Autodesk Inventor part; units mm, degrees
(part 3 of 3)
  line L1410 (3.7715, -2.9179) -> (3.7996, -2.8422)
  line L1411 (3.7996, -2.8422) -> (3.7715, -2.9179)
  line L1412 (3.747, -2.9958) -> (3.7715, -2.9179)
  line L1413 (3.7715, -2.9179) -> (3.747, -2.9958)
  line L1414 (3.7261, -3.0758) -> (3.747, -2.9958)
  line L1415 (3.747, -2.9958) -> (3.7261, -3.0758)
  line L1416 (3.7095, -3.158) -> (3.7261, -3.0758)
  line L1417 (3.7261, -3.0758) -> (3.7095, -3.158)
  line L1418 (3.6965, -3.2424) -> (3.7095, -3.158)
  line L1419 (3.7095, -3.158) -> (3.6965, -3.2424)
  line L1420 (3.6879, -3.3289) -> (3.6965, -3.2424)
  line L1421 (3.6965, -3.2424) -> (3.6879, -3.3289)
  line L1422 (3.6828, -3.4176) -> (3.6879, -3.3289)
  line L1423 (3.6879, -3.3289) -> (3.6828, -3.4176)
  line L1424 (3.6814, -3.4911) -> (3.6828, -3.4176)
  line L1425 (3.6828, -3.4176) -> (3.6814, -3.4911)
  line L1426 (3.6843, -3.5899) -> (3.6814, -3.4911)
  line L1427 (3.6814, -3.4911) -> (3.6843, -3.5899)
  line L1428 (3.6944, -3.6821) -> (3.6843, -3.5899)
  line L1429 (3.6843, -3.5899) -> (3.6944, -3.6821)
  line L1430 (3.7102, -3.7687) -> (3.6944, -3.6821)
  line L1431 (3.6944, -3.6821) -> (3.7102, -3.7687)
  line L1432 (3.7326, -3.848) -> (3.7102, -3.7687)
  line L1433 (3.7102, -3.7687) -> (3.7326, -3.848)
  line L1434 (3.7607, -3.9215) -> (3.7326, -3.848)
  line L1435 (3.7326, -3.848) -> (3.7607, -3.9215)
  line L1436 (3.796, -3.9893) -> (3.7607, -3.9215)
  line L1437 (3.7607, -3.9215) -> (3.796, -3.9893)
  line L1438 (3.8371, -4.0498) -> (3.796, -3.9893)
  line L1439 (3.796, -3.9893) -> (3.8371, -4.0498)
  line L1440 (3.8796, -4.0989) -> (3.8371, -4.0498)
  line L1441 (3.8371, -4.0498) -> (3.8796, -4.0989)
  line L1442 (3.9366, -4.1515) -> (3.8796, -4.0989)
  line L1443 (3.8796, -4.0989) -> (3.9366, -4.1515)
  line L1444 (4, -4.1962) -> (3.9366, -4.1515)
  line L1445 (3.9366, -4.1515) -> (4, -4.1962)
  line L1446 (4.0693, -4.2337) -> (4, -4.1962)
  line L1447 (4, -4.1962) -> (4.0693, -4.2337)
  line L1448 (4.1435, -4.2625) -> (4.0693, -4.2337)
  line L1449 (4.0693, -4.2337) -> (4.1435, -4.2625)
  line L1450 (4.2235, -4.2841) -> (4.1435, -4.2625)
  line L1451 (4.1435, -4.2625) -> (4.2235, -4.2841)
  line L1452 (4.3101, -4.2978) -> (4.2235, -4.2841)
  line L1453 (4.2235, -4.2841) -> (4.3101, -4.2978)
  line L1454 (4.4016, -4.3036) -> (4.3101, -4.2978)
  line L1455 (4.3101, -4.2978) -> (4.4016, -4.3036)
  line L1456 (4.4268, -4.3043) -> (4.4016, -4.3036)
  line L1457 (4.4016, -4.3036) -> (4.4268, -4.3043)
  line L1458 (5.4867, -4.2863) -> (5.7138, -3.1998)
  line L1459 (5.7138, -3.1998) -> (5.4867, -4.2863)
  line L1460 (5.4174, -4.3274) -> (5.4867, -4.2863)
  line L1461 (5.4867, -4.2863) -> (5.4174, -4.3274)
  line L1462 (4.5011, -4.3014) -> (4.4268, -4.3043)
  line L1463 (4.4268, -4.3043) -> (4.5011, -4.3014)
  line L1464 (4.5768, -4.2935) -> (4.5011, -4.3014)
  line L1465 (4.5011, -4.3014) -> (4.5768, -4.2935)
  line L1466 (4.6539, -4.2805) -> (4.5768, -4.2935)
  line L1467 (4.5768, -4.2935) -> (4.6539, -4.2805)
  line L1468 (4.7318, -4.2625) -> (4.6539, -4.2805)
  line L1469 (4.6539, -4.2805) -> (4.7318, -4.2625)
  line L1470 (4.8111, -4.2394) -> (4.7318, -4.2625)
  line L1471 (4.7318, -4.2625) -> (4.8111, -4.2394)
  line L1472 (4.8919, -4.2106) -> (4.8111, -4.2394)
  line L1473 (4.8111, -4.2394) -> (4.8919, -4.2106)
  line L1474 (4.9733, -4.1767) -> (4.8919, -4.2106)
  line L1475 (4.8919, -4.2106) -> (4.9733, -4.1767)
  line L1476 (5.0562, -4.1378) -> (4.9733, -4.1767)
  line L1477 (4.9733, -4.1767) -> (5.0562, -4.1378)
  line L1478 (5.1406, -4.0938) -> (5.0562, -4.1378)
  line L1479 (5.0562, -4.1378) -> (5.1406, -4.0938)
  line L1480 (5.1738, -4.0751) -> (5.1406, -4.0938)
  line L1481 (5.1406, -4.0938) -> (5.1738, -4.0751)
  line L1482 (5.2942, -3.5019) -> (5.1738, -4.0751)
  line L1483 (5.1738, -4.0751) -> (5.2942, -3.5019)
  line L1484 (4.4831, -3.5019) -> (5.2942, -3.5019)
  line L1485 (5.2942, -3.5019) -> (4.4831, -3.5019)
  line L1486 (4.5465, -3.1998) -> (4.4831, -3.5019)
  line L1487 (4.4831, -3.5019) -> (4.5465, -3.1998)
  line L1488 (5.7138, -3.1998) -> (4.5465, -3.1998)
  line L1489 (4.5465, -3.1998) -> (5.7138, -3.1998)
  line L1490 (5.6229, -2.1984) -> (5.5717, -2.1379)
  line L1491 (5.5717, -2.1379) -> (5.6229, -2.1984)
  line L1492 (5.6373, -2.2179) -> (5.6229, -2.1984)
  line L1493 (5.6229, -2.1984) -> (5.6373, -2.2179)
  line L1494 (5.677, -2.2813) -> (5.6373, -2.2179)
  line L1495 (5.6373, -2.2179) -> (5.677, -2.2813)
  line L1496 (5.713, -2.3513) -> (5.677, -2.2813)
  line L1497 (5.677, -2.2813) -> (5.713, -2.3513)
  line L1498 (5.7448, -2.427) -> (5.713, -2.3513)
  line L1499 (5.713, -2.3513) -> (5.7448, -2.427)
  line L1500 (5.7721, -2.5092) -> (5.7448, -2.427)
  line L1501 (5.7448, -2.427) -> (5.7721, -2.5092)
  line L1502 (5.7952, -2.5978) -> (5.7721, -2.5092)
  line L1503 (5.7721, -2.5092) -> (5.7952, -2.5978)
  line L1504 (5.8104, -2.667) -> (5.7952, -2.5978)
  line L1505 (5.7952, -2.5978) -> (5.8104, -2.667)
  line L1506 (5.4614, -2.7053) -> (5.8104, -2.667)
  line L1507 (5.8104, -2.667) -> (5.4614, -2.7053)
  line L1508 (5.4383, -2.6159) -> (5.4614, -2.7053)
  line L1509 (5.4614, -2.7053) -> (5.4383, -2.6159)
  line L1510 (5.4088, -2.5337) -> (5.4383, -2.6159)
  line L1511 (5.4383, -2.6159) -> (5.4088, -2.5337)
  line L1512 (5.3727, -2.4587) -> (5.4088, -2.5337)
  line L1513 (5.4088, -2.5337) -> (5.3727, -2.4587)
  line L1514 (5.3288, -2.3909) -> (5.3727, -2.4587)
  line L1515 (5.3727, -2.4587) -> (5.3288, -2.3909)
  line L1516 (5.279, -2.3304) -> (5.3288, -2.3909)
  line L1517 (5.3288, -2.3909) -> (5.279, -2.3304)
  line L1518 (5.2285, -2.2835) -> (5.279, -2.3304)
  line L1519 (5.279, -2.3304) -> (5.2285, -2.2835)
  line L1520 (5.1644, -2.2381) -> (5.2285, -2.2835)
  line L1521 (5.2285, -2.2835) -> (5.1644, -2.2381)
  line L1522 (5.0952, -2.2013) -> (5.1644, -2.2381)
  line L1523 (5.1644, -2.2381) -> (5.0952, -2.2013)
  line L1524 (5.0195, -2.1725) -> (5.0952, -2.2013)
  line L1525 (5.0952, -2.2013) -> (5.0195, -2.1725)
  line L1526 (4.9387, -2.1523) -> (5.0195, -2.1725)
  line L1527 (5.0195, -2.1725) -> (4.9387, -2.1523)
  line L1528 (4.8515, -2.1407) -> (4.9387, -2.1523)
  line L1529 (4.9387, -2.1523) -> (4.8515, -2.1407)
  line L1530 (4.7722, -2.1379) -> (4.8515, -2.1407)
  line L1531 (4.8515, -2.1407) -> (4.7722, -2.1379)
  line L1532 (20, -5.5833) -> (20.6667, -0.5833)
  line L1533 (20, -5.5833) -> (20.6667, -0.5833)
  line L1534 (-20.6667, -5.5833) -> (20, -5.5833)
  line L1535 (-20.6667, -5.5833) -> (20, -5.5833)
  line L1536 (-20, -0.5833) -> (-20.6667, -5.5833)
  line L1537 (-20, -0.5833) -> (-20.6667, -5.5833)
  line L1538 (20.6667, -0.5833) -> (-20, -0.5833)
  line L1539 (20.6667, -0.5833) -> (-20, -0.5833)
  line L1540 (15.8547, -2.1761) -> (15.9643, -2.1797)
  line L1541 (15.9643, -2.1797) -> (15.8547, -2.1761)
  line L1542 (15.9643, -2.1797) -> (16.0551, -2.1869)
  line L1543 (16.0551, -2.1869) -> (15.9643, -2.1797)
  line L1544 (16.0551, -2.1869) -> (16.1265, -2.1984)
  line L1545 (16.1265, -2.1984) -> (16.0551, -2.1869)
  line L1546 (16.1265, -2.1984) -> (16.1799, -2.2143)
  line L1547 (16.1799, -2.2143) -> (16.1265, -2.1984)
  line L1548 (16.1799, -2.2143) -> (16.2022, -2.2251)
  line L1549 (16.2022, -2.2251) -> (16.1799, -2.2143)
  line L1550 (16.2022, -2.2251) -> (16.2707, -2.2727)
  line L1551 (16.2707, -2.2727) -> (16.2022, -2.2251)
  line L1552 (16.2707, -2.2727) -> (16.3233, -2.3361)
  line L1553 (16.3233, -2.3361) -> (16.2707, -2.2727)
  line L1554 (16.3233, -2.3361) -> (16.3457, -2.3801)
  line L1555 (16.3457, -2.3801) -> (16.3233, -2.3361)
  line L1556 (16.3457, -2.3801) -> (16.3673, -2.4587)
  line L1557 (16.3673, -2.4587) -> (16.3457, -2.3801)
  line L1558 (16.3673, -2.4587) -> (16.3745, -2.551)
  line L1559 (16.3745, -2.551) -> (16.3673, -2.4587)
  line L1560 (16.3745, -2.551) -> (16.3745, -2.5539)
  line L1561 (16.3745, -2.5539) -> (16.3745, -2.551)
  line L1562 (16.3745, -2.5539) -> (16.368, -2.6368)
  line L1563 (16.368, -2.6368) -> (16.3745, -2.5539)
  line L1564 (16.368, -2.6368) -> (16.35, -2.7168)
  line L1565 (16.35, -2.7168) -> (16.368, -2.6368)
  line L1566 (16.35, -2.7168) -> (16.3197, -2.7947)
  line L1567 (16.3197, -2.7947) -> (16.35, -2.7168)
  line L1568 (16.3197, -2.7947) -> (16.2779, -2.8711)
  line L1569 (16.2779, -2.8711) -> (16.3197, -2.7947)
  line L1570 (16.2779, -2.8711) -> (16.2729, -2.879)
  line L1571 (16.2729, -2.879) -> (16.2779, -2.8711)
  line L1572 (16.2729, -2.879) -> (16.221, -2.9468)
  line L1573 (16.221, -2.9468) -> (16.2729, -2.879)
  line L1574 (16.221, -2.9468) -> (16.1618, -3.0052)
  line L1575 (16.1618, -3.0052) -> (16.221, -2.9468)
  line L1576 (16.1618, -3.0052) -> (16.0955, -3.0549)
  line L1577 (16.0955, -3.0549) -> (16.1618, -3.0052)
  line L1578 (16.0955, -3.0549) -> (16.0212, -3.0946)
  line L1579 (16.0212, -3.0946) -> (16.0955, -3.0549)
  line L1580 (16.0212, -3.0946) -> (16.0191, -3.096)
  line L1581 (16.0191, -3.096) -> (16.0212, -3.0946)
  line L1582 (16.0191, -3.096) -> (15.9607, -3.1184)
  line L1583 (15.9607, -3.1184) -> (16.0191, -3.096)
  line L1584 (15.9607, -3.1184) -> (15.8922, -3.1364)
  line L1585 (15.8922, -3.1364) -> (15.9607, -3.1184)
  line L1586 (15.8922, -3.1364) -> (15.8143, -3.1508)
  line L1587 (15.8143, -3.1508) -> (15.8922, -3.1364)
  line L1588 (15.8143, -3.1508) -> (15.7257, -3.1609)
  line L1589 (15.7257, -3.1609) -> (15.8143, -3.1508)
  line L1590 (15.7257, -3.1609) -> (15.6276, -3.1674)
  line L1591 (15.6276, -3.1674) -> (15.7257, -3.1609)
  line L1592 (15.6276, -3.1674) -> (15.5195, -3.1688)
  line L1593 (15.5195, -3.1688) -> (15.6276, -3.1674)
  line L1594 (15.5195, -3.1688) -> (14.9326, -3.1688)
  line L1595 (14.9326, -3.1688) -> (15.5195, -3.1688)
  line L1596 (14.9326, -3.1688) -> (15.1395, -2.1761)
  line L1597 (15.1395, -2.1761) -> (14.9326, -3.1688)
  line L1598 (15.1395, -2.1761) -> (15.8547, -2.1761)
  line L1599 (15.8547, -2.1761) -> (15.1395, -2.1761)
  line L1600 (15.1395, -2.1761) -> (15.8547, -2.1761)
  line L1601 (15.8547, -2.1761) -> (15.9643, -2.1797)
  line L1602 (15.9643, -2.1797) -> (16.0551, -2.1869)
  line L1603 (16.0551, -2.1869) -> (16.1265, -2.1984)
  line L1604 (16.1265, -2.1984) -> (16.1799, -2.2143)
  line L1605 (16.1799, -2.2143) -> (16.2022, -2.2251)
  line L1606 (16.2022, -2.2251) -> (16.2707, -2.2727)
  line L1607 (16.2707, -2.2727) -> (16.3233, -2.3361)
  line L1608 (16.3233, -2.3361) -> (16.3457, -2.3801)
  line L1609 (16.3457, -2.3801) -> (16.3673, -2.4587)
  line L1610 (16.3673, -2.4587) -> (16.3745, -2.551)
  line L1611 (16.3745, -2.551) -> (16.3745, -2.5539)
  line L1612 (16.3745, -2.5539) -> (16.368, -2.6368)
  line L1613 (16.368, -2.6368) -> (16.35, -2.7168)
  line L1614 (16.35, -2.7168) -> (16.3197, -2.7947)
  line L1615 (16.3197, -2.7947) -> (16.2779, -2.8711)
  line L1616 (16.2779, -2.8711) -> (16.2729, -2.879)
  line L1617 (16.2729, -2.879) -> (16.221, -2.9468)
  line L1618 (16.221, -2.9468) -> (16.1618, -3.0052)
  line L1619 (16.1618, -3.0052) -> (16.0955, -3.0549)
  line L1620 (16.0955, -3.0549) -> (16.0212, -3.0946)
  line L1621 (16.0212, -3.0946) -> (16.0191, -3.096)
  line L1622 (16.0191, -3.096) -> (15.9607, -3.1184)
  line L1623 (15.9607, -3.1184) -> (15.8922, -3.1364)
  line L1624 (15.8922, -3.1364) -> (15.8143, -3.1508)
  line L1625 (15.8143, -3.1508) -> (15.7257, -3.1609)
  line L1626 (15.7257, -3.1609) -> (15.6276, -3.1674)
  line L1627 (15.6276, -3.1674) -> (15.5195, -3.1688)
  line L1628 (15.5195, -3.1688) -> (14.9326, -3.1688)
  line L1629 (14.9326, -3.1688) -> (15.1395, -2.1761)
  line L1630 (15.8547, -2.1761) -> (15.1395, -2.1761)
  line L1631 (15.1395, -2.1761) -> (14.9326, -3.1688)
  line L1632 (14.9326, -3.1688) -> (15.5195, -3.1688)
  line L1633 (15.5195, -3.1688) -> (15.6276, -3.1674)
  line L1634 (15.6276, -3.1674) -> (15.7257, -3.1609)
  line L1635 (15.7257, -3.1609) -> (15.8143, -3.1508)
  line L1636 (15.8143, -3.1508) -> (15.8922, -3.1364)
  line L1637 (15.8922, -3.1364) -> (15.9607, -3.1184)
  line L1638 (15.9607, -3.1184) -> (16.0191, -3.096)
  line L1639 (16.0191, -3.096) -> (16.0212, -3.0946)
  line L1640 (16.0212, -3.0946) -> (16.0955, -3.0549)
  line L1641 (16.0955, -3.0549) -> (16.1618, -3.0052)
  line L1642 (16.1618, -3.0052) -> (16.221, -2.9468)
  line L1643 (16.221, -2.9468) -> (16.2729, -2.879)
  line L1644 (16.2729, -2.879) -> (16.2779, -2.8711)
  line L1645 (16.2779, -2.8711) -> (16.3197, -2.7947)
  line L1646 (16.3197, -2.7947) -> (16.35, -2.7168)
  line L1647 (16.35, -2.7168) -> (16.368, -2.6368)
  line L1648 (16.368, -2.6368) -> (16.3745, -2.5539)
  line L1649 (16.3745, -2.5539) -> (16.3745, -2.551)
  line L1650 (16.3745, -2.551) -> (16.3673, -2.4587)
  line L1651 (16.3673, -2.4587) -> (16.3457, -2.3801)
  line L1652 (16.3457, -2.3801) -> (16.3233, -2.3361)
  line L1653 (16.3233, -2.3361) -> (16.2707, -2.2727)
  line L1654 (16.2707, -2.2727) -> (16.2022, -2.2251)
  line L1655 (16.2022, -2.2251) -> (16.1799, -2.2143)
  line L1656 (16.1799, -2.2143) -> (16.1265, -2.1984)
  line L1657 (16.1265, -2.1984) -> (16.0551, -2.1869)
  line L1658 (16.0551, -2.1869) -> (15.9643, -2.1797)
  line L1659 (15.9643, -2.1797) -> (15.8547, -2.1761)
  arc A47 (-2.261, -3.2608) -> (-2.1774, -2.3167) centre (-2.277, -2.7836) ccw
  line L1660 (-2.6757, -2.3167) -> (-2.1774, -2.3167)
  line L1661 (-2.261, -3.2608) -> (-2.8422, -3.2608)
  line L1662 (-2.8422, -3.2608) -> (-2.261, -3.2608)
  line L1663 (-12.4787, -3.1906) -> (-12.3602, -2.9373)
  line L1664 (-12.3602, -2.9373) -> (-12.4787, -3.1906)
  line L1665 (-12.3602, -2.9373) -> (-12.1495, -2.7468)
  line L1666 (-12.1495, -2.7468) -> (-12.3602, -2.9373)
  line L1667 (-12.1495, -2.7468) -> (-11.8819, -2.6358)
  line L1668 (-11.8819, -2.6358) -> (-12.1495, -2.7468)
  arc A48 (-11.5251, -2.6521) -> (-11.8819, -2.6358) centre (-11.7304, -3.23) ccw
  arc A49 (-11.5251, -2.6521) -> (-11.8819, -2.6358) centre (-11.7304, -3.23) ccw
  arc A50 (-11.1823, -3.2751) -> (-11.5251, -2.6521) centre (-11.7466, -3.1798) ccw
  arc A51 (-11.1823, -3.2751) -> (-11.5251, -2.6521) centre (-11.7466, -3.1798) ccw
  arc A52 (-11.9452, -4.0358) -> (-11.1823, -3.2751) centre (-11.983, -3.235) ccw
  arc A53 (-11.9452, -4.0358) -> (-11.1823, -3.2751) centre (-11.983, -3.235) ccw
  arc A54 (-12.5101, -3.3677) -> (-11.9452, -4.0358) centre (-11.9452, -3.463) ccw
  arc A55 (-12.5101, -3.3677) -> (-11.9452, -4.0358) centre (-11.9452, -3.463) ccw
  line L1669 (-12.5101, -3.3677) -> (-12.4787, -3.1906)
  line L1670 (-12.4787, -3.1906) -> (-12.5101, -3.3677)
  line L1671 (-12.5101, -3.3677) -> (-12.4787, -3.1906)
  line L1672 (-12.4787, -3.1906) -> (-12.3602, -2.9373)
  line L1673 (-12.3602, -2.9373) -> (-12.1495, -2.7468)
  line L1674 (-12.1495, -2.7468) -> (-11.8819, -2.6358)
  arc A56 (-11.5251, -2.6521) -> (-11.8819, -2.6358) centre (-11.7304, -3.23) ccw
  arc A57 (-11.1823, -3.2751) -> (-11.5251, -2.6521) centre (-11.7466, -3.1798) ccw
  arc A58 (-11.9452, -4.0358) -> (-11.1823, -3.2751) centre (-11.983, -3.235) ccw
  arc A59 (-12.5101, -3.3677) -> (-11.9452, -4.0358) centre (-11.9452, -3.463) ccw
  line L1675 (-12.4787, -3.1906) -> (-12.5101, -3.3677)
  arc A60 (-12.5101, -3.3677) -> (-11.9452, -4.0358) centre (-11.9452, -3.463) ccw
  arc A61 (-11.9452, -4.0358) -> (-11.1823, -3.2751) centre (-11.983, -3.235) ccw
  arc A62 (-11.1823, -3.2751) -> (-11.5251, -2.6521) centre (-11.7466, -3.1798) ccw
  arc A63 (-11.5251, -2.6521) -> (-11.8819, -2.6358) centre (-11.7304, -3.23) ccw
  line L1676 (-11.8819, -2.6358) -> (-12.1495, -2.7468)
  line L1677 (-12.1495, -2.7468) -> (-12.3602, -2.9373)
  line L1678 (-12.3602, -2.9373) -> (-12.4787, -3.1906)
  arc A64 (-15.2153, -4.2591) -> (-15.2122, -3.2293) centre (-15.2303, -3.7441) ccw
  line L1679 (-15.4912, -1.9003) -> (-15.6491, -2.8294)
  line L1680 (-15.7237, -3.2293) -> (-15.2122, -3.2293)
  line L1681 (-15.9053, -4.2591) -> (-15.2153, -4.2591)
  line L1682 (-15.7237, -3.2293) -> (-15.9053, -4.2591)
  line L1683 (-2.6757, -2.3167) -> (-2.8422, -3.2608)
  point P0 (0, 0)
  point P1 (-14.2731, -2.9167)
  point P2 (-13.78, -3.5707)
  point P3 (-14.2731, -2.9167)
  point P4 (-13.78, -3.5707)
  point P5 (-1.4506, -3.3546)
  point P6 (-1.4506, -3.3546)
  point P7 (-0.2619, -2.715)
  point P8 (-0.2619, -2.715)
  point P9 (1.3891, -3.9863)
  point P10 (1.3891, -3.9863)
  point P11 (-11.5251, -2.6521)
  point P12 (-11.5251, -2.6521)
  point P13 (-11.1823, -3.2751)
  point P14 (-11.1823, -3.2751)
  point P15 (-11.9452, -4.0358)
  point P16 (-11.9452, -4.0358)
  point P17 (-15.2122, -3.2293)
sketch "Sketch10" plane through (0, 0, 0) normal (0, 1, 0) x (-1, 0, 0)
  line L0 (10, 10) -> (-10, 10)
  line L1 (-10, 10) -> (-10, -10)
  line L2 (-10, -10) -> (10, -10)
  line L3 (10, -10) -> (10, 10)
  line L4 (10, 10) -> (-10, -10) construction
  line L5 (-10, 10) -> (10, -10) construction
  point P0 (0, 0)
  dimension "d33" = 20
  dimension "d34" = 20
  constraints: 12 end point, 2 midpoint, 2 parallel, 1 horizontal, 1 perpendicular
  measures "d33" distance between parallel lines of L0 L2
  measures "d34" distance between parallel lines of L1 L3
extrude "Extrusion4" add sketch "Sketch10" along normal mid plane 20
body "Solid4"
